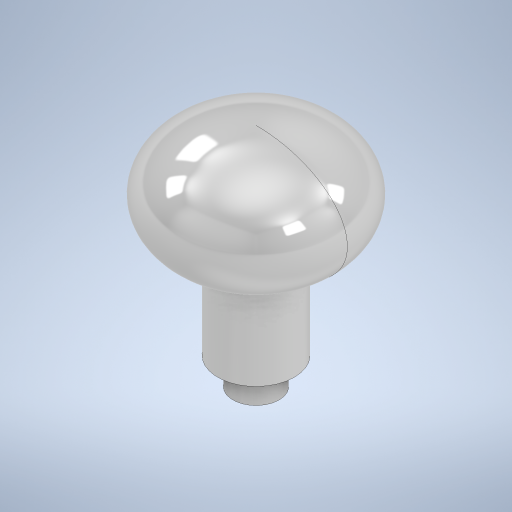
# Autodesk Inventor part: PMT_
Saved by Autodesk Inventor 2023 (Build 270158000, 158)
## iProperties
Created: 2022-05-16
Part Number: PMT_
Material: Stainless Steel
Document SubType Name: Modeling
Designer: 50255
Density: 8 g/cm^3
Appearance: Aluminum - Dark
Author: 50255
Autodesk Inventor part; units mm, degrees
ref_plane "YZ Plane" through (0, 0, 0) normal (1, 0, 0) x (0, 1, 0)
ref_plane "XZ Plane" through (0, 0, 0) normal (0, 1, 0) x (-1, 0, 0)
ref_plane "XY Plane" through (0, 0, 0) normal (0, 0, 1) x (1, 0, 0)
sketch "Sketch1" plane through (0, 0, 0) normal (0, 0, 1) x (1, 0, 0)
  line L0 (0, 0) -> (25.6, 0)
  line L1 (25.6, 0) -> (25.6, 30)
  line L2 (25.6, 30) -> (42.25, 30)
  line L3 (42.25, 30) -> (42.25, 85.5975)
  arc A0 (55.2402, 129.665) -> (42.25, 119) centre (66.8347, 102.2988) ccw
  ellipse E0 centre (0, 184.5) end of major axis (0, 250) minor radius 101 (55.2402, 129.665) -> (0, 250) ccw
  line L4 (42.25, 85.5975) -> (42.25, 119)
  line L5 (0, 184.5) -> (101, 184.5) construction
  line L6 (0, 206.73) -> (95.0052, 206.73) construction
  line L7 (0, 0) -> (0, 250)
  dimension "d15" = 101
  dimension "d0" = 25.6
  dimension "d1" = 30
  dimension "d2" = 16.65
  dimension "d16" = 95.0053
  dimension "d17" = 250
  constraints: 16 end point, 4 horizontal, 4 vertical, 3 point on circle, 1 centre point, 6 other
  measures "d0" distance of L0.start L0.end
  measures "d1" distance of L0.end L1.end
  measures "d2" distance of L1.end L2.end
  measures "d16" distance of L6.start L6.end
  measures "d17" distance of L0.start L7.end
sketch "Sketch3" plane through (0, 0, 0) normal (0, 0, 1) x (1, 0, 0)
  point P0 (0, 0)
revolve "Revolution2" add sketch "Sketch1" angle 360 about axis through (0, 0, 0) along (0, 1, 0)
body "Solid2"
